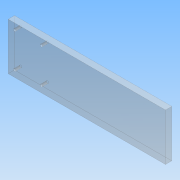
# Autodesk Inventor part: Luna_base
Saved by Autodesk Inventor 2016 (Build 200138000, 138)
## iProperties
Created: 2015-08-03
Part Number: Luna_base
Material: Generic
Document SubType Name: Modeling
Designer: Openlab
Density: 1 g/cm^3
Appearance: Polycarbonate - Clear
Author: Openlab
Autodesk Inventor part; units mm, degrees
ref_plane "YZ Plane" through (0, 0, 0) normal (1, 0, 0) x (0, 1, 0)
ref_plane "XZ Plane" through (0, 0, 0) normal (0, 1, 0) x (-1, 0, 0)
ref_plane "XY Plane" through (0, 0, 0) normal (0, 0, 1) x (1, 0, 0)
sketch "Sketch1" plane through (0, 0, 0) normal (0, 1, 0) x (-1, 0, 0)
  line L0 (0, 0) -> (200, 0)
  line L1 (200, 0) -> (200, -60)
  line L2 (200, -60) -> (0, -60)
  line L3 (0, -60) -> (0, 0)
  dimension "d0" = 200
  dimension "d1" = 60
  constraints: 8 end point, 2 parallel, 1 horizontal, 1 perpendicular
  measures "d0" distance of L1.end L2.end
  measures "d1" distance of L0.end L1.end
extrude "Extrusion1" add sketch "Sketch1" along normal blind 8
sketch "Sketch2" plane through (0, 8, 0) normal (0, 1, 0) x (1, 0, 0)
  line L0 (-155, 55) -> (-155, 5)
  line L1 (-160, 17.25) -> (-160, 25.75)
  line L2 (-160, 25.75) -> (-161, 25.75)
  line L3 (-161, 25.75) -> (-161, 17.25)
  line L4 (-161, 17.25) -> (-160, 17.25)
  line L5 (-161, 34.25) -> (-160, 34.25)
  line L6 (-160, 34.25) -> (-160, 42.75)
  line L7 (-160, 42.75) -> (-161, 42.75)
  line L8 (-161, 42.75) -> (-161, 34.25)
  line L9 (-155, 55) -> (-195, 55)
  line L10 (-195, 5) -> (-155, 5)
  line L11 (-127.49, 30) -> (-133.3125, 30) construction
  line L12 (-195, 5) -> (-195, 55)
  circle A0 centre (-158, 52) radius 1.5
  circle A1 centre (-192, 52) radius 1.5
  circle A2 centre (-158, 8) radius 1.5
  circle A3 centre (-192, 8) radius 1.5
  line L13 (-200, 60) -> (-200, 0) projected
  line L14 (-200, 0) -> (0, 0) projected
  point P0 (-159.5, 47)
  point P1 (-159.5, 30)
  point P2 (-159.5, 13)
  dimension "d4" = 8.5
  dimension "d5" = 1
  dimension "d6" = 5
  dimension "d7" = 17
  dimension "d8" = 17
  dimension "d9" = 4.25
  dimension "d10" = 4.25
  dimension "d11" = 4.5
  dimension "d12" = 40
  dimension "d13" = 50
  dimension "d14" = 3
  dimension "d15" = 3
  dimension "d16" = 3
  dimension "d17" = 3
  dimension "d18" = 3
  dimension "d19" = 5
  dimension "d20" = 5
  constraints: 26 end point, 6 perpendicular, 4 centre point, 4 coincident, 4 vertical alignment, 3 equal radius, 2 equal length, 2 horizontal, 2 horizontal alignment, 2 parallel, 2 point on line, 1 collinear, 1 vertical, 1 other
  measures "d4" distance of L7.end L5.start
  measures "d5" distance of L6.end L7.end
  measures "d6" distance between parallel lines of L0 L6
  measures "d7" distance of point (-159.5, 30) point (-159.5, 47)
  measures "d8" distance of point (-159.5, 13) point (-159.5, 30)
  measures "d9" distance from line of L7 point (-159.5, 47)
  measures "d10" distance from line of point (-159.5, 30) L2
  measures "d11" distance from line of L0 point (-159.5, 13)
  measures "d12" distance of L0.start L9.end
  measures "d13" distance of L0.start L0.end
  measures "d14" diameter of A0
  measures "d15" distance from line of L0 A0.centre
  measures "d16" distance from line of L9 A0.centre
  measures "d17" distance from line of L10 A3.centre
  measures "d18" distance from line of L12 A3.centre
  measures "d19" distance between parallel lines of L12 L13
  measures "d20" distance between parallel lines of L14 L10
hole "Hole1" at (-158, 8, -8) at (-158, 8, -52) at (-192, 8, -52) at (-192, 8, -8) direction (0, -1, 0) diameter 3 end through all
body "Solid1"
